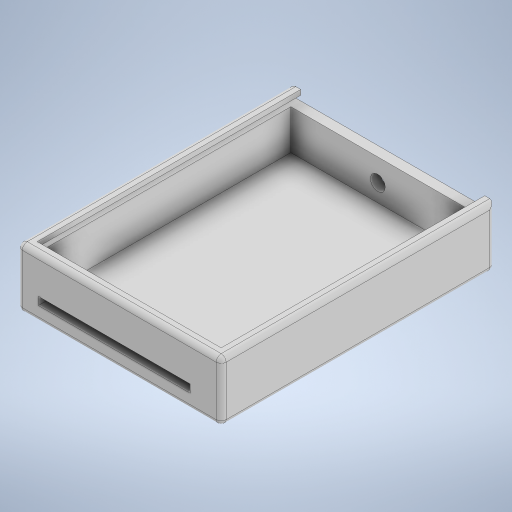
# Autodesk Inventor part: case_basic
Saved by Autodesk Inventor 2024 (Build 280153000, 153)
## iProperties
Created: 2024-02-17
Part Number: case_basic
Material: 一般
Document SubType Name: Modeling
Designer: Akio
Density: 1 g/cm^3
Appearance: 既定
Author: Akio
Autodesk Inventor part; units mm, degrees
ref_plane "YZ Plane" through (0, 0, 0) normal (1, 0, 0) x (0, 1, 0)
ref_plane "XZ Plane" through (0, 0, 0) normal (0, 1, 0) x (-1, 0, 0)
ref_plane "XY Plane" through (0, 0, 0) normal (0, 0, 1) x (1, 0, 0)
sketch "スケッチ1" plane through (0, 0, 0) normal (0, 1, 0) x (-1, 0, 0)
  line L0 (0, 0) -> (-41, 0)
  line L1 (-41, 0) -> (-41, -55)
  line L2 (-41, -55) -> (0, -55)
  line L3 (0, -55) -> (0, 0)
  dimension "d0" = 41
  dimension "d1" = 55
  constraints: 8 end point, 2 parallel, 1 horizontal, 1 perpendicular
  measures "d0" distance of L2.end L1.end
  measures "d1" distance of L1.end L0.end
extrude "押し出し1" add sketch "スケッチ1" along normal blind 12
sketch "スケッチ3" plane through (0, 12, 0) normal (0, 1, 0) x (1, 0, 0)
  line L0 (2, 2) -> (39, 2)
  line L1 (39, 2) -> (39, 53)
  line L2 (39, 53) -> (2, 53)
  line L3 (2, 53) -> (2, 2)
  line L4 (0, 55) -> (0, 0) projected
  line L5 (0, 0) -> (41, 0) projected
  dimension "d4" = 37
  dimension "d5" = 51
  dimension "d6" = 2
  dimension "d7" = 2
  constraints: 8 end point, 2 parallel, 1 horizontal, 1 perpendicular
  measures "d4" distance of L2.end L1.end
  measures "d5" distance of L1.end L0.end
  measures "d6" distance between parallel lines of L4 L3
  measures "d7" distance between parallel lines of L5 L0
extrude "押し出し2" cut sketch "スケッチ3" against normal blind 10
sketch "スケッチ4" plane through (0, 0, 0) normal (0, 0, 1) x (1, 0, 0)
  line L0 (4.25, 4.6) -> (34.75, 4.6)
  line L1 (34.75, 4.6) -> (34.75, 3)
  line L2 (34.75, 3) -> (4.25, 3)
  line L3 (4.25, 3) -> (4.25, 4.6)
  line L4 (0, 0) -> (41, 0) projected
  line L5 (0, 0) -> (0, 12) projected
  point P0 (4.25, 3.8)
  point P1 (19.5, 4.6)
  dimension "d10" = 30.5
  dimension "d11" = 1.6
  dimension "d12" = 3
  dimension "d14" = 19.5
  constraints: 8 end point, 2 midpoint, 2 parallel, 1 horizontal, 1 perpendicular
  measures "d10" distance of L1.end L2.end
  measures "d11" distance of L0.end L1.end
  measures "d12" distance between parallel lines of L4 L2
  measures "d14" distance from line of L5 point (19.5, 4.6)
extrude "押し出し3" cut sketch "スケッチ4" against normal blind 10
sketch "スケッチ5" plane through (41, 0, -55) normal (0, 0, -1) x (-1, 0, 0)
  circle A0 centre (21.5, 5.5) radius 1.5
  line L0 (41, 0) -> (41, 12) projected
  line L1 (0, 12) -> (41, 12) projected
  dimension "d17" = 3
  dimension "d18" = 19.5
  dimension "d19" = 6.5
  constraints: 1 centre point
  measures "d17" diameter of A0
  measures "d18" distance from line of L0 A0.centre
  measures "d19" distance from line of A0.centre L1
extrude "押し出し4" cut sketch "スケッチ5" against normal blind 10
sketch "スケッチ7" plane through (41, 0, -55) normal (0, 0, -1) x (-1, 0, 0)
  line L0 (40, 11) -> (1, 11)
  line L1 (1, 11) -> (1, 10)
  line L2 (1, 10) -> (40, 10)
  line L3 (40, 10) -> (40, 11)
  line L4 (41, 0) -> (41, 12) projected
  line L5 (0, 12) -> (41, 12) projected
  point P0 (20.5, 10)
  dimension "d22" = 39
  dimension "d23" = 1
  dimension "d24" = 20.5
  dimension "d25" = 1
  constraints: 8 end point, 2 parallel, 1 horizontal, 1 midpoint, 1 perpendicular
  measures "d22" distance of L2.end L1.end
  measures "d23" distance of L1.end L0.end
  measures "d24" distance from line of L4 point (20.5, 10)
  measures "d25" distance between parallel lines of L5 L0
extrude "押し出し5" cut sketch "スケッチ7" against normal blind 54
sketch "スケッチ8" plane through (41, 0, -55) normal (0, 0, -1) x (-1, 0, 0)
  line L0 (39, 12) -> (2, 12)
  line L1 (2, 12) -> (2, 11)
  line L2 (2, 11) -> (39, 11)
  line L3 (39, 11) -> (39, 12)
  line L4 (41, 0) -> (41, 12) projected
  line L5 (0, 12) -> (41, 12) projected
  point P0 (20.5, 12)
  dimension "d28" = 37
  dimension "d29" = 1
  dimension "d30" = 20.5
  dimension "d31" = 0
  constraints: 8 end point, 2 parallel, 1 horizontal, 1 midpoint, 1 perpendicular
  measures "d28" distance of L2.end L1.end
  measures "d29" distance of L1.end L0.end
  measures "d30" distance from line of L4 point (20.5, 12)
  measures "d31" distance between parallel lines of L5 L0
extrude "押し出し6" cut sketch "スケッチ8" against normal blind 2
fillet "フィレット1" radius 1 11 edges at (0, 6, 0) (41, 6, 0) (20.5, 12, 0) (41, 12, -27.5) (20.5, 0, -55) (0, 6, -55) (0, 0, -27.5) (20.5, 0, 0) (41, 0, -27.5) (41, 6, -55) (0, 12, -27.5)
